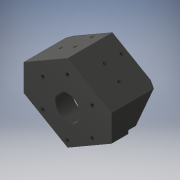
# Autodesk Inventor part: BO12
Saved by Autodesk Inventor 2017 (Build 210142000, 142)
## iProperties
Created: 2018-10-22
Part Number: BO12
Material: ABS Plastic
Document SubType Name: Modeling
Designer: Dell
Density: 1.06 g/cm^3
Appearance: Smooth - Black
Author: Dell
Autodesk Inventor part; units mm, degrees
ref_plane "YZ Plane" through (0, 0, 0) normal (1, 0, 0) x (0, 1, 0)
ref_plane "XZ Plane" through (0, 0, 0) normal (0, 1, 0) x (-1, 0, 0)
ref_plane "XY Plane" through (0, 0, 0) normal (0, 0, 1) x (1, 0, 0)
sketch "Sketch1" plane through (0, 0, 0) normal (0, 0, 1) x (1, 0, 0)
  line L0 (0, 0) -> (0, 104.428)
  line L1 (0, 104.428) -> (-48.4974, 76.428)
  line L2 (-48.4974, 76.428) -> (-48.4974, 0)
  line L3 (-48.4974, 0) -> (48.4974, 0)
  line L4 (48.4974, 0) -> (48.4974, 76.428)
  line L5 (48.4974, 76.428) -> (0, 104.428)
  line L6 (0, -28) -> (-48.4974, 0)
  line L7 (-48.4974, 0) -> (-48.4974, 56)
  line L8 (-48.4974, 56) -> (0, 84)
  line L9 (0, 84) -> (48.4974, 56)
  line L10 (48.4974, 56) -> (48.4974, 0)
  line L11 (48.4974, 0) -> (0, -28)
  circle A0 centre (0, -23) radius 3
  circle A1 centre (44.1673, 2.5) radius 3
  circle A2 centre (44.1673, 53.5) radius 3
  circle A3 centre (0, 79) radius 3
  circle A4 centre (-44.1673, 53.5) radius 3
  circle A5 centre (-44.1673, 2.5) radius 3
  line L12 (48.4974, 76.428) -> (48.4974, 56)
  line L13 (48.4974, 56) -> (0, 84)
  line L14 (0, 84) -> (-48.4974, 56)
  line L15 (-48.4974, 56) -> (-48.4974, 76.428)
  point P0 (0, 28)
  dimension "d1" = 60
  dimension "d2" = 60
  dimension "d43" = 112
  dimension "d44" = 76.4279
  dimension "d45" = 6
  dimension "d46" = 5
  dimension "d49" = 360
  constraints: 32 end point, 6 centre point, 3 collinear, 3 vertical, 2 perpendicular, 2 point on line, 1 midpoint, 1 vertical alignment, 26 other
  measures "d1" angle of L0 L5
  measures "d2" angle of L1 L0
  measures "d43" distance of L6.start L8.end
  measures "d44" distance of point (0, 28) L0.end
  measures "d45" diameter of A0
  measures "d46" distance of L6.start A0.centre
extrude "Extrusion1" add sketch "Sketch1" along normal blind 10 contours L8 L2 L1 L0 | L9 L4 L3 A1 L0 A3 | L0 A3 L3 A5 L2 L8 | L0 L5 L4 L9 | L3 A5 A1 L11 L6
sketch "Sketch2" plane through (0, 0, 0) normal (0, 0, -1) x (-1, 0, 0)
  line L0 (0, 104.428) -> (48.4974, 76.428)
  line L1 (-48.4974, 76.428) -> (0, 104.428)
  line L2 (48.4974, 76.428) -> (48.4974, 0) construction
  line L3 (-48.4974, 0) -> (-48.4974, 76.428) construction
  line L4 (-48.4974, 64.8809) -> (0, 92.8809)
  line L5 (0, 92.8809) -> (48.4974, 64.8809)
  line L6 (48.4974, 76.428) -> (48.4974, 0)
  line L7 (-48.4974, 64.8809) -> (-48.4974, 76.428)
  line L8 (0, 104.428) -> (48.4974, 76.428)
  line L9 (48.4974, 64.8809) -> (48.4974, 76.428)
  line L10 (-48.4974, 0) -> (-48.4974, 76.428)
  line L11 (48.4974, 76.428) -> (48.4974, 0)
  line L12 (-48.4974, 0) -> (-48.4974, 76.428) projected
  point P0 (-48.4974, 38.214)
  point P1 (48.4974, 38.214)
  dimension "d7" = 10
  constraints: 24 end point, 4 coincident, 4 midpoint, 3 point on line, 2 parallel, 1 collinear, 1 vertical, 1 vertical alignment
  measures "d7" distance between parallel lines of L1 L4
extrude "Extrusion2" add sketch "Sketch2" along normal blind 50
sketch "Sketch3" plane through (0, 92.8809, -50) normal (-0.5, -0.8660254, 0) x (0.8660254, -0.5, 0)
  circle A0 centre (28, 25) radius 2.5
  line L0 (56, 50) -> (56, 0) projected
  line L1 (56, 0) -> (0, 0) projected
  point P0 (46.4405, 50)
  point P1 (28, 0)
  point P2 (56, 25)
  dimension "d10" = 5
  constraints: 2 midpoint, 1 centre point, 1 horizontal alignment, 1 vertical alignment
  measures "d10" diameter of A0
extrude "Extrusion3" cut sketch "Sketch3" against normal through all
sketch "Sketch4" plane through (-48.4974, 64.8809, -50) normal (0.5, -0.8660254, 0) x (0.8660254, 0.5, 0)
  line L0 (0, 50) -> (0, 0) projected
  line L1 (56, 0) -> (0, 0) projected
  circle A0 centre (28, 25) radius 2.5
  point P0 (9.5595, 50)
  point P1 (28, 0)
  point P2 (0, 25)
  dimension "d13" = 5
  constraints: 2 midpoint, 1 centre point, 1 horizontal alignment, 1 vertical alignment
  measures "d13" diameter of A0
extrude "Extrusion4" cut sketch "Sketch4" against normal through all
sketch "Sketch10" plane through (0, 0, 0) normal (0, 0, -1) x (-1, 0, 0)
  circle A0 centre (0, 79) radius 3 construction
  circle A1 centre (0, -23) radius 3 construction
  line L0 (0, -23) -> (0, 79) construction
  circle A2 centre (0, 28) radius 22.5
  point P0 (0, 0)
  dimension "d51" = 45
  constraints: 2 end point, 1 centre point, 1 midpoint, 1 vertical
  measures "d51" diameter of A2
extrude "Extrusion9" cut sketch "Sketch10" against normal through all
sketch "Sketch11" plane through (-48.4974, 0, 10) normal (-1, 0, 0) x (0, 0, 1)
  line L0 (-60, 76.428) -> (-60, 64.8809) projected
  line L1 (-60, 64.8809) -> (-60, 76.428)
  line L2 (0, 76.428) -> (-60, 76.428) projected
  line L3 (-60, 76.428) -> (0, 76.428)
  line L4 (0, 76.428) -> (0, 0) projected
  line L5 (0, 76.428) -> (0, 0)
  line L6 (-10, 0) -> (0, 0) projected
  line L7 (0, 0) -> (-10, 0)
  line L8 (-10, -0.5) -> (-10, 5.5) projected
  line L9 (-10, 0) -> (0, 0) projected
  line L10 (-60, 64.8809) -> (-10, 0)
  constraints: 10 end point, 3 collinear, 1 perpendicular
extrude "Extrusion10" add sketch "Sketch11" along normal blind 30
sketch "Sketch12" plane through (48.4974, 0, 10) normal (1, 0, 0) x (0, 0, -1)
  line L0 (10, 0) -> (0, 0) projected
  line L1 (0, 0) -> (0, 76.428) projected
  line L2 (0, 76.428) -> (60, 76.428) projected
  line L3 (60, 76.428) -> (60, 64.8809) projected
  line L4 (60, 64.8809) -> (10, 0) projected
  point P0 (10, 0)
extrude "Extrusion11" add sketch "Sketch12" along normal blind 30
sketch "Sketch13" plane through (0, 0, 0) normal (0, 0, -1) x (-1, 0, 0)
  circle A0 centre (-44.1673, 53.5) radius 3 construction
  circle A1 centre (-44.1673, 53.5) radius 6.5
  circle A2 centre (0, 28) radius 22.5 construction
  circle A3 centre (-44.1673, 2.5) radius 6.5
  circle A4 centre (0, -23) radius 6.5
  circle A5 centre (44.1673, 2.5) radius 6.5
  circle A6 centre (44.1673, 53.5) radius 6.5
  circle A7 centre (0, 79) radius 6.5
  point P0 (0, 0)
  dimension "d58" = 13
  dimension "d61" = 360
  constraints: 6 centre point, 1 coincident, 13 other
  measures "d58" diameter of A1
extrude "Extrusion12" cut sketch "Sketch13" along normal through all
sketch "Sketch14" plane through (0, 0, 10) normal (0, 0, 1) x (1, 0, 0)
  line L0 (48.4974, 76.428) -> (0, 104.428) projected
  line L1 (48.4974, 76.428) -> (78.4974, 59.1074)
  line L2 (78.4974, 64.8809) -> (78.4974, 76.428) projected
  line L3 (78.4974, 59.1074) -> (78.4974, 76.428)
  line L4 (48.4974, 76.428) -> (78.4974, 76.428) projected
  line L5 (48.4974, 76.428) -> (78.4974, 76.428)
  line L6 (0, 0) -> (0, 104.428)
  line L7 (-48.4974, 76.428) -> (-78.4974, 59.1074)
  line L8 (-78.4974, 64.8809) -> (-78.4974, 76.428)
  line L9 (-78.4974, 59.1074) -> (-78.4974, 76.428)
  line L10 (-48.4974, 76.428) -> (-78.4974, 76.428)
  line L11 (-48.4974, 76.428) -> (-78.4974, 76.428)
  constraints: 18 end point, 4 symmetric about line, 3 collinear, 2 point on line, 1 vertical
extrude "Extrusion13" cut sketch "Sketch14" against normal through all
sketch "Sketch15" plane through (0, 0, 0) normal (0, 0, -1) x (-1, 0, 0)
  line L0 (0, -28) -> (-48.4974, 0) projected
  line L1 (0, -28) -> (-91.9808, 25.1051)
  line L2 (-91.9808, 25.1051) -> (-91.9808, -28)
  line L3 (-91.9808, -28) -> (0, -28)
  line L4 (0, -28) -> (91.276, 24.6982)
  line L5 (91.276, 24.6982) -> (91.276, -28)
  line L6 (48.4974, 0) -> (0, -28) projected
  line L7 (91.276, -28) -> (0, -28)
  line L8 (48.4974, 0) -> (0, -28) projected
  point P0 (0, 0)
  point P1 (24.2487, -14)
  point P2 (24.2487, -14)
  constraints: 12 end point, 3 midpoint, 3 perpendicular, 2 point on line, 1 collinear, 1 vertical
extrude "Extrusion14" cut sketch "Sketch15" along normal through all both and the other way through all
sketch "Sketch16" plane through (0, 0, 10) normal (0, 0, 1) x (1, 0, 0)
  line L0 (0, -28) -> (78.4974, 17.3205) projected
  line L1 (78.4974, 17.3205) -> (78.4974, 11.547)
  line L2 (78.4974, 11.547) -> (0, -33.7735)
  line L3 (0, -33.7735) -> (-78.4974, 11.547)
  line L4 (-78.4974, 64.8809) -> (-78.4974, 17.3205) projected
  line L5 (-78.4974, 11.547) -> (-78.4974, 17.3205)
  line L6 (-78.4974, 17.3205) -> (0, -28) projected
  point P0 (0, 0)
  dimension "d69" = 5
  constraints: 8 end point, 2 parallel, 2 vertical, 1 vertical alignment
  measures "d69" distance between parallel lines of L0 L2
extrude "Extrusion15" add sketch "Sketch16" against normal blind 10
sketch "Sketch18" plane through (0, 0, 0) normal (0, 0, -1) x (-1, 0, 0)
  line L0 (-48.4974, 64.8809) -> (0, 92.8809) projected
  line L1 (0, 92.8809) -> (48.4974, 64.8809) projected
  line L2 (-38.4974, 47.5604) -> (0, 69.7869)
  line L3 (0, 69.7869) -> (38.4974, 47.5604)
  line L4 (-38.4974, 47.5604) -> (-48.4974, 41.7869)
  line L5 (-48.4974, 7.3477) -> (-48.4974, 48.6523) projected
  line L6 (38.4974, 47.5604) -> (48.4974, 41.7869)
  line L7 (48.4974, 48.6523) -> (48.4974, 7.3477) projected
  circle A0 centre (-44.1673, 53.5) radius 3 projected
  circle A1 centre (0, 79) radius 3 projected
  circle A2 centre (44.1673, 53.5) radius 3 projected
  circle A3 centre (-44.1673, 53.5) radius 6.5
  circle A4 centre (0, 79) radius 6.5
  circle A5 centre (44.1673, 53.5) radius 6.5
  line L8 (-48.4974, 41.7869) -> (-48.4974, 48.6523)
  line L9 (-48.4974, 64.8809) -> (-48.4974, 58.3477) projected
  line L10 (-48.4974, 58.3477) -> (-48.4974, 64.8809)
  line L11 (0, 92.8809) -> (-48.4974, 64.8809) projected
  line L12 (-48.4974, 64.8809) -> (0, 92.8809)
  line L13 (0, 92.8809) -> (48.4974, 64.8809)
  line L14 (48.4974, 64.8809) -> (48.4974, 58.3477) projected
  line L15 (48.4974, 64.8809) -> (48.4974, 58.3477)
  line L16 (48.4974, 41.7869) -> (48.4974, 48.6523)
  arc A6 (-48.4974, 58.3477) -> (-48.4974, 48.6523) centre (-44.1673, 53.5) ccw
  arc A7 (48.4974, 48.6523) -> (48.4974, 58.3477) centre (44.1673, 53.5) ccw
  point P0 (0, 0)
  dimension "d72" = 20
  dimension "d73" = 13
  constraints: 20 end point, 7 collinear, 4 point on circle, 3 centre point, 3 coincident, 2 point on line, 8 other
  measures "d72" distance between parallel lines of L0 L2
  measures "d73" diameter of A4
extrude "Extrusion16" add sketch "Sketch18" along normal blind 50 contours L0 L1 L14 A5 L7 L6 L3 L2 L4 L5 A3 L9
sketch "Sketch19" plane through (-48.4974, 41.7869, -50) normal (-1, 0, 0) x (0, 0, 1)
  line L0 (12.5065, 6.8654) -> (17.7972, 0) projected
  line L1 (12.5065, 6.8654) -> (0, 6.8654) projected
  line L2 (0, 0) -> (0, 6.8654) projected
  line L3 (17.7972, 0) -> (0, 0) projected
  line L4 (0, 23.094) -> (5.0348, 16.5607) projected
  line L5 (0, 16.5607) -> (0, 23.094) projected
  line L6 (5.0348, 16.5607) -> (0, 16.5607) projected
  line L7 (0, 16.5607) -> (0, 6.8654)
  line L8 (12.5065, 6.8654) -> (5.0348, 16.5607) projected
  line L9 (5.0348, 16.5607) -> (12.5065, 6.8654)
  point P0 (50, -41.7869)
  constraints: 4 end point, 1 collinear, 1 perpendicular
extrude "Extrusion17" cut sketch "Sketch19" against normal through all
sketch "Sketch20" plane through (0, 69.7869, -50) normal (-0.5, -0.8660254, 0) x (0.8660254, -0.5, 0)
  circle A0 centre (43, 40) radius 2.5
  circle A1 centre (13, 40) radius 2.5
  circle A2 centre (13, 10) radius 2.5
  line L0 (43, 40) -> (13, 40) construction
  line L1 (13, 10) -> (13, 40) construction
  line L2 (13, 10) -> (43, 40) construction
  line L3 (0, 50) -> (56, 50) projected
  point P0 (34.8935, 50)
  point P1 (28, 40)
  point P2 (28, 50)
  dimension "d78" = 5
  dimension "d79" = 5
  dimension "d80" = 5
  dimension "d81" = 45
  dimension "d83" = 30
  dimension "d84" = 10
  constraints: 6 end point, 3 centre point, 2 midpoint, 1 coincident, 1 horizontal, 1 vertical, 1 vertical alignment
  measures "d78" diameter of A0
  measures "d79" diameter of A1
  measures "d80" diameter of A2
  measures "d81" angle of L0 L2
  measures "d83" distance of L0.start L0.end
  measures "d84" distance between parallel lines of L3 L0
extrude "Extrusion18" cut sketch "Sketch20" against normal through all
sketch "Sketch21" plane through (0, 104.428, 10) normal (0.5, 0.8660254, 0) x (0.8660254, -0.5, 0)
  circle A0 centre (33.7735, 35) radius 2.5 projected
  point P0 (52.214, 10)
extrude "Extrusion19" add sketch "Sketch21" against normal blind 10
mirror "Mirror2" about plane through (0, 0, 0) normal (1, 0, 0) of "Extrusion18"
mirror "Mirror3" about plane through (0, 0, 0) normal (1, 0, 0) of "Extrusion19"
sketch "Sketch23" plane through (0, 0, 10) normal (0, 0, 1) x (1, 0, 0)
  line L0 (78.4974, 59.1074) -> (78.4974, 11.547) projected
  line L1 (78.4974, 59.1074) -> (0, 104.428) projected
  line L2 (0, 104.428) -> (-78.4974, 59.1074) projected
  line L3 (-78.4974, 11.547) -> (-78.4974, 59.1074) projected
  line L4 (0, -33.7735) -> (-78.4974, 11.547) projected
  line L5 (78.4974, 11.547) -> (0, -33.7735) projected
  circle A0 centre (0, 28) radius 22.5 projected
  circle A1 centre (-44.1673, 53.5) radius 3 projected
  circle A2 centre (44.1673, 53.5) radius 3 projected
  circle A3 centre (-44.1673, 2.5) radius 3 projected
  circle A4 centre (0, 79) radius 3 projected
  circle A5 centre (44.1673, 2.5) radius 3 projected
  circle A6 centre (0, -23) radius 3 projected
  point P0 (0, 0)
extrude "Extrusion20" add sketch "Sketch23" along normal blind 20
body "Solid1"
